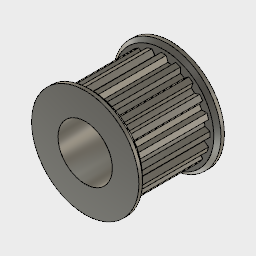
squaretoothpulley (Autodesk Fusion 360 design; units mm, degrees)
Autodesk Fusion 360 part; units mm, degrees
sketch "Sketch1" plane through (0, 0, 0) normal (0, 1, 0) x (1, 0, 0)
  circle A0 centre (0, 0) radius 3.81
  circle A1 centre (0, 0) radius 5.81
  dimension "shaftDiameter" = 7.62
  dimension "outerDiameter" = 11.62
  constraint concentric A0 A1
  measures "shaftDiameter" diameter of A0
  measures "outerDiameter" diameter of A1
extrude "Extrude1" add sketch "Sketch1" along normal blind 10 contours A0 | A1
sketch "Sketch2" plane through (0, 0, 0) normal (0, -1, 0) x (1, 0, 0)
  circle A0 centre (0, 0) radius 5.81
  circle A1 centre (0, 0) radius 7.53
  circle A2 centre (0, 0) radius 3.81
  dimension "flangeDiameter" = 15.06
  dimension "d25" = 7.62
  constraint concentric A1 A2
  measures "flangeDiameter" diameter of A1
  measures "d25" diameter of A2
extrude "Extrude2" add sketch "Sketch2" along normal blind 1 contours A0 | A1 | A2
sketch "Sketch3" plane through (0, 10, 0) normal (0, 1, 0) x (-1, 0, 0)
  circle A0 centre (0, 0) radius 5.81
  circle A1 centre (0, 0) radius 3.81
  circle A2 centre (0, 0) radius 7.53
  dimension "d9" = 7.62
  dimension "d10" = 15.06
  constraint concentric A1 A2
  measures "d9" diameter of A1
  measures "d10" diameter of A2
extrude "Extrude3" add sketch "Sketch3" along normal blind 1 contours A0 | A1 | A2
sketch "Sketch4" plane through (0, 0, 0) normal (0, 1, 0) x (-1, 0, 0)
  circle A0 centre (0, 0) radius 7.53
  circle A1 centre (0, 0) radius 5.81
  circle A2 centre (0, 0) radius 5.81
  line L0 (-0.5939, 5.7796) -> (-0.36, 6.4996)
  line L1 (-0.36, 6.4996) -> (0.36, 6.4996)
  line L2 (0.36, 6.4996) -> (0.5939, 5.7796)
  circle A3 centre (0, 0) radius 5.81
  dimension "d13" = 11.62
  dimension "d14" = 108
  dimension "d15" = 108
  dimension "toothWidth" = 0.72
  dimension "d17" = 0.36
  dimension "toothHeight" = 0.72
  constraint concentric A0 A1
  constraint coincident A1
  constraint horizontal L1
  constraint coincident A2
  measures "d13" diameter of A1
  measures "d14" angle of L1 L2
  measures "d15" angle of L0 L1
extrude "Extrude4" add sketch "Sketch4" along normal up to surface (10 mm away) contours A1 A2 L0 L1 L2 A3
pattern_circular "C-Pattern1" count 20 over 360 about axis through (0, 1.75, 0) along (0, 1, 0) of "Extrude4"
chamfer "Chamfer1" distance 0.5 angle 45 2 edges at (-7.0204, 0, -2.723) (7.0204, 10, -2.723)
hole "Hole1" at (0, 11, 0) direction (0, -1, 0) diameter 7.62 end up to surface (12 mm away)
equation "outerDiameter = shaftDiameter + 4 mm"
equation "flangeDiameter = outerDiameter + ( 2 * toothHeight ) + 2 mm"
equation "d9 = shaftDiameter"
equation "d10 = flangeDiameter"
equation "d13 = outerDiameter"
equation "toothWidth = ( 1.2 * 12 / 7.62 ) * shaftDiameter / teethNum"
equation "d17 = toothWidth / 2"
equation "toothHeight = ( toothWidth / 7.62 mm ) * shaftDiameter"
equation "d20 = teethNum"
equation "teethNum = 20"
equation "d25 = shaftDiameter"
equation "d28 = shaftDiameter"
